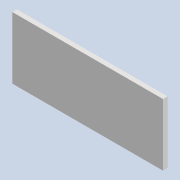
# Autodesk Inventor part: 00_Baseplate_Simmo_side5_v2
Saved by Autodesk Inventor 2022 (Build 260153000, 153)
## iProperties
Created: 2022-08-09
Part Number: 00_Baseplate_Simmo_side5_v2
Material: Generic
Document SubType Name: Modeling
Designer: wanghaoran
Density: 1 g/cm^3
Appearance: Default
Author: wanghaoran
Autodesk Inventor part; units mm, degrees
ref_plane "YZ Plane" through (0, 0, 0) normal (1, 0, 0) x (0, 1, 0)
ref_plane "XZ Plane" through (0, 0, 0) normal (0, 1, 0) x (-1, 0, 0)
ref_plane "XY Plane" through (0, 0, 0) normal (0, 0, 1) x (1, 0, 0)
sketch "Sketch1" plane through (0, 0, 0) normal (0, 0, 1) x (1, 0, 0)
  line L0 (184.3024, 0) -> (184.3024, 6) projected
  line L1 (-10, 0) -> (-10, 6) projected
  line L2 (184.3024, 6) -> (0, 6)
  line L3 (0, 6) -> (0, -74)
  line L4 (0, -74) -> (184.3024, -74)
  line L5 (184.3024, -74) -> (184.3024, 6)
  line L6 (-10, 6) -> (0, 6)
  line L7 (0, 6) -> (0, -74)
  line L8 (0, -74) -> (-10, -74)
  line L9 (-10, -74) -> (-10, 6)
  point P0 (0, 0)
  dimension "d0" = 80
  constraints: 16 end point, 4 parallel, 2 horizontal, 2 perpendicular
  measures "d0" distance of L3.end L2.end
extrude "Extrusion1" add sketch "Sketch1" along normal blind 6
sketch "Sketch4" plane through (0, 0, 6) normal (0, 0, 1) x (1, 0, 0)
  line L0 (160, 0) -> (184.3024, 0) projected
  line L1 (160, 6) -> (160, 0) projected
  line L2 (184.3024, 6) -> (-10, 6) projected
  line L3 (184.3024, -74) -> (184.3024, 6) projected
  line L4 (0, 0) -> (-10, 0) projected
  line L5 (0, 6) -> (0, 0) projected
  line L6 (-10, 6) -> (-10, -74) projected
extrude "Extrusion4" cut sketch "Sketch4" against normal blind 6 contours L1 L2 L3 L0
sketch "Sketch5" plane through (0, 0, 6) normal (0, 0, 1) x (1, 0, 0)
  line L0 (140, 0) -> (150, 0) projected
  line L1 (150, 0) -> (150, 6) projected
  line L2 (140, 6) -> (140, 0) projected
  line L3 (160, 6) -> (-10, 6) projected
  line L4 (150, 0) -> (150.1, 0)
  line L5 (150.1, 0) -> (150.1, 6)
  line L6 (150.1, 6) -> (150, 6)
  line L7 (150, 6) -> (150, 0)
  line L8 (140, 0) -> (139.9, 0)
  line L9 (139.9, 0) -> (139.9, 6)
  line L10 (139.9, 6) -> (140, 6)
  line L11 (140, 6) -> (140, 0)
  point P0 (0, 0)
  point P1 (0, 6)
  dimension "d21" = 0.1
  dimension "d22" = 6
  dimension "d23" = 0.1
  dimension "d24" = 6
  constraints: 16 end point, 4 parallel, 2 horizontal, 2 perpendicular
  measures "d21" distance of L6.end L5.end
  measures "d22" distance of L5.end L4.end
  measures "d23" distance of L9.end L10.end
  measures "d24" distance of L8.end L9.end
extrude "Extrusion5" cut sketch "Sketch5" against normal blind 6
pattern_linear "Rectangular Pattern3" count 8 spacing 20 along (-1, 0, 0) of "Extrusion5"
ref_plane "Work Plane1" through (-10, -34, 0) normal (0, -1, 0) x (1, 0, 0)
mirror "Mirror1" about plane through (-10, -34, 0) normal (0, -1, 0) of "Extrusion5"
pattern_linear "Rectangular Pattern4" count 2 spacing 20 along (1, 0, 0) count 8 spacing 20 along (-1, 0, 0) of "Extrusion5", "Mirror1"
sketch "Sketch6" plane through (0, 0, 6) normal (0, 0, 1) x (1, 0, 0)
  line L0 (167.75, -4.4) -> (162.25, -4.4)
  line L1 (162.25, -4.4) -> (162.25, -2)
  line L2 (162.25, -2) -> (167.75, -2)
  line L3 (167.75, -2) -> (167.75, -4.4)
  line L4 (159.9, 0) -> (159.9, 6) projected
  line L5 (184.3024, 0) -> (159.9, 0) projected
  line L6 (147.75, -4.4) -> (142.25, -4.4)
  line L7 (142.25, -4.4) -> (142.25, -2)
  line L8 (142.25, -2) -> (147.75, -2)
  line L9 (147.75, -2) -> (147.75, -4.4)
  line L10 (150.1, 0) -> (139.9, 0) projected
  line L11 (139.9, 0) -> (139.9, 6) projected
  point P0 (0, 0)
  dimension "d36" = 5.5
  dimension "d37" = 2.4
  dimension "d38" = 2.35
  dimension "d39" = 2
  dimension "d48" = 5.5
  dimension "d49" = 2.4
  dimension "d50" = 2
  dimension "d51" = 2.35
  constraints: 16 end point, 4 parallel, 2 horizontal, 2 perpendicular
  measures "d36" distance of L1.end L2.end
  measures "d37" distance of L0.end L1.end
  measures "d38" distance between parallel lines of L4 L1
  measures "d39" distance between parallel lines of L5 L2
  measures "d48" distance of L7.end L8.end
  measures "d49" distance of L6.end L7.end
  measures "d50" distance between parallel lines of L10 L8
  measures "d51" distance between parallel lines of L11 L7
extrude "Extrusion6" cut sketch "Sketch6" against normal blind 6 contours L6 L7 L8 L9
pattern_linear "Rectangular Pattern5" count 3 spacing 60 along (-1, 0, 0) count 2 spacing 61.6 along (0, -1, 0) of "Extrusion6"
body "Solid1"
